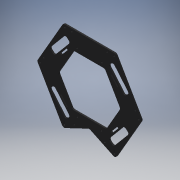
# Autodesk Inventor part: Bottom Plate
Saved by Autodesk Inventor 2017 (Build 210142000, 142)
## iProperties
Created: 2016-10-01
Part Number: Bottom Plate
Material: PVC, Unplasticized
Document SubType Name: Modeling
Designer: James Yelland
Density: 1.29 g/cm^3
Appearance: Smooth - White
Mass: 37.5584 g
Surface Area: 327.952 cm^2
Volume: 29.115 cm^3
Author: James Yelland
Autodesk Inventor part; units mm, degrees
ref_plane "YZ Plane" through (0, 0, 0) normal (1, 0, 0) x (0, 1, 0)
ref_plane "XZ Plane" through (0, 0, 0) normal (0, 1, 0) x (-1, 0, 0)
ref_plane "XY Plane" through (0, 0, 0) normal (0, 0, 1) x (1, 0, 0)
sketch "Sketch1" plane through (0, 0, 0) normal (0, 1, 0) x (-1, 0, 0)
  line L0 (103.5566, -2.5) -> (54.8095, -86.9325)
  line L1 (-54.8095, -86.9325) -> (-103.5566, -2.5)
  line L2 (-103.5566, 2.5) -> (-53.9434, 88.4327)
  line L3 (-49.6132, 90.9327) -> (49.6132, 90.9327)
  line L4 (53.9434, 88.4327) -> (103.5566, 2.5)
  line L5 (2.1497, -66.9563) -> (48.3297, -88.9468)
  line L6 (-2.1497, -66.9563) -> (-48.3297, -88.9468)
  arc A0 (48.3297, -88.9468) -> (54.8095, -86.9325) centre (50.4794, -84.4325) ccw
  arc A1 (2.1497, -66.9563) -> (-2.1497, -66.9563) centre (0, -71.4706) ccw
  arc A2 (-54.8095, -86.9325) -> (-48.3297, -88.9468) centre (-50.4794, -84.4325) ccw
  arc A3 (-103.5566, 2.5) -> (-103.5566, -2.5) centre (-99.2265, 0) ccw
  arc A4 (-49.6132, 90.9327) -> (-53.9434, 88.4327) centre (-49.6132, 85.9327) ccw
  arc A5 (53.9434, 88.4327) -> (49.6132, 90.9327) centre (49.6132, 85.9327) ccw
  arc A6 (103.5566, -2.5) -> (103.5566, 2.5) centre (99.2265, 0) ccw
  circle A7 centre (49.6132, 85.9327) radius 1.6
  circle A8 centre (-49.6132, 85.9327) radius 1.6
  circle A9 centre (-99.2265, 0) radius 1.6
  circle A10 centre (99.2265, 0) radius 1.6
  circle A11 centre (-25, 62.282) radius 1.6
  circle A12 centre (25, 62.282) radius 1.6
  circle A13 centre (24, -57.282) radius 1.6
  circle A14 centre (-24, -57.282) radius 1.6
  circle A15 centre (-30.6147, -73.9104) radius 1.6
  circle A16 centre (30.6147, -73.9104) radius 1.6
  circle A17 centre (35.5991, 85.9437) radius 1.6
  circle A18 centre (-35.5945, 85.9327) radius 1.6
  circle A19 centre (92.2171, 12.1406) radius 1.6
  circle A20 centre (-92.2171, 12.1406) radius 1.6
  arc A21 (31.3397, -49.282) -> (35.6699, -46.782) centre (31.3397, -44.282) ccw
  line L7 (31.3397, -49.282) -> (-31.3397, -49.282)
  arc A22 (-35.6699, -46.782) -> (-31.3397, -49.282) centre (-31.3397, -44.282) ccw
  line L8 (-35.6699, -46.782) -> (-61.2361, -2.5)
  arc A23 (-61.2361, 2.5) -> (-61.2361, -2.5) centre (-56.906, 0) ccw
  line L9 (-61.2361, 2.5) -> (-32.7831, 51.782)
  arc A24 (-28.453, 54.282) -> (-32.7831, 51.782) centre (-28.453, 49.282) ccw
  line L10 (-28.453, 54.282) -> (28.453, 54.282)
  arc A25 (32.7831, 51.782) -> (28.453, 54.282) centre (28.453, 49.282) ccw
  line L11 (32.7831, 51.782) -> (61.2361, 2.5)
  arc A26 (61.2361, -2.5) -> (61.2361, 2.5) centre (56.906, 0) ccw
  line L12 (61.2361, -2.5) -> (35.6699, -46.782)
  arc A27 (67.8361, 29.5077) -> (73.4714, 29.0147) centre (70.9003, 32.0789) ccw
  arc A28 (77.3017, 32.2286) -> (77.7947, 37.8639) centre (74.7305, 35.2928) ccw
  line L13 (73.4714, 29.0147) -> (77.3017, 32.2286)
  arc A29 (50.7976, 70.0378) -> (45.1623, 70.5308) centre (47.7335, 67.4666) ccw
  line L14 (45.1623, 70.5308) -> (41.3321, 67.3169)
  arc A30 (41.3321, 67.3169) -> (40.8391, 61.6815) centre (43.9032, 64.2527) ccw
  line L15 (64.2962, 53.9509) -> (50.7976, 70.0378)
  line L16 (64.2962, 53.9509) -> (77.7947, 37.8639)
  line L17 (40.8391, 61.6815) -> (67.8361, 29.5077)
  line L18 (49.7796, 41.77) -> (43.3517, 49.4305)
  line L19 (43.3517, 49.4305) -> (45.6499, 51.3589)
  line L20 (45.6499, 51.3589) -> (58.5056, 36.038)
  line L21 (58.5056, 36.038) -> (56.2075, 34.1096)
  line L22 (56.2075, 34.1096) -> (49.7796, 41.77)
  arc A31 (73.4714, -29.0147) -> (67.8361, -29.5077) centre (70.9003, -32.0789) ccw
  line L23 (54.3376, -45.5946) -> (57.5515, -41.7644)
  line L24 (45.6499, -51.3589) -> (58.5056, -36.038)
  line L25 (58.5056, -36.038) -> (56.2075, -34.1096)
  line L26 (40.8391, -61.6815) -> (67.8361, -29.5077)
  line L27 (64.2962, -53.9509) -> (77.7947, -37.8639)
  line L28 (73.4714, -29.0147) -> (77.3017, -32.2286)
  arc A32 (77.7947, -37.8639) -> (77.3017, -32.2286) centre (74.7305, -35.2928) ccw
  line L29 (43.3517, -49.4305) -> (45.6499, -51.3589)
  line L30 (49.7796, -41.77) -> (43.3517, -49.4305)
  arc A33 (45.1623, -70.5308) -> (50.7976, -70.0378) centre (47.7335, -67.4666) ccw
  line L31 (64.2962, -53.9509) -> (50.7976, -70.0378)
  line L32 (45.1623, -70.5308) -> (41.3321, -67.3169)
  arc A34 (40.8391, -61.6815) -> (41.3321, -67.3169) centre (43.9032, -64.2527) ccw
  line L33 (56.2075, -34.1096) -> (49.7796, -41.77)
  line L34 (-40.8391, -61.6815) -> (-67.8361, -29.5077)
  arc A35 (-67.8361, -29.5077) -> (-73.4714, -29.0147) centre (-70.9003, -32.0789) ccw
  line L35 (-45.6499, -51.3589) -> (-58.5056, -36.038)
  line L36 (-64.2962, -53.9509) -> (-77.7947, -37.8639)
  line L37 (-73.4714, -29.0147) -> (-77.3017, -32.2286)
  arc A36 (-77.3017, -32.2286) -> (-77.7947, -37.8639) centre (-74.7305, -35.2928) ccw
  line L38 (-43.3517, -49.4305) -> (-45.6499, -51.3589)
  line L39 (-49.7796, -41.77) -> (-43.3517, -49.4305)
  line L40 (-56.2075, -34.1096) -> (-49.7796, -41.77)
  line L41 (-45.1623, -70.5308) -> (-41.3321, -67.3169)
  arc A37 (-50.7976, -70.0378) -> (-45.1623, -70.5308) centre (-47.7335, -67.4666) ccw
  line L42 (-64.2962, -53.9509) -> (-50.7976, -70.0378)
  arc A38 (-41.3321, -67.3169) -> (-40.8391, -61.6815) centre (-43.9032, -64.2527) ccw
  line L43 (-40.8391, 61.6815) -> (-67.8361, 29.5077)
  arc A39 (-73.4714, 29.0147) -> (-67.8361, 29.5077) centre (-70.9003, 32.0789) ccw
  line L44 (-73.4714, 29.0147) -> (-77.3017, 32.2286)
  arc A40 (-77.7947, 37.8639) -> (-77.3017, 32.2286) centre (-74.7305, 35.2928) ccw
  line L45 (-64.2962, 53.9509) -> (-77.7947, 37.8639)
  line L46 (-56.2075, 34.1096) -> (-49.7796, 41.77)
  line L47 (-49.7796, 41.77) -> (-43.3517, 49.4305)
  line L48 (-45.6499, 51.3589) -> (-58.5056, 36.038)
  line L49 (-58.5056, 36.038) -> (-56.2075, 34.1096)
  line L50 (-64.2962, 53.9509) -> (-50.7976, 70.0378)
  line L51 (-43.3517, 49.4305) -> (-45.6499, 51.3589)
  line L52 (-45.1623, 70.5308) -> (-41.3321, 67.3169)
  arc A41 (-45.1623, 70.5308) -> (-50.7976, 70.0378) centre (-47.7335, 67.4666) ccw
  arc A42 (-40.8391, 61.6815) -> (-41.3321, 67.3169) centre (-43.9032, 64.2527) ccw
  line L53 (51.9794, -77.4325) -> (51.9794, -85.4325)
  line L54 (51.9794, -85.4325) -> (48.9794, -85.4325)
  line L55 (48.9794, -85.4325) -> (48.9794, -77.4325)
  line L56 (48.9794, -77.4325) -> (51.9794, -77.4325)
  line L57 (-48.9794, -77.4325) -> (-48.9794, -85.4325)
  line L58 (-48.9794, -85.4325) -> (-51.9794, -85.4325)
  line L59 (-51.9794, -85.4325) -> (-51.9794, -77.4325)
  line L60 (-51.9794, -77.4325) -> (-48.9794, -77.4325)
  line L61 (-56.2075, -34.1096) -> (-58.5056, -36.038)
  point P0 (52.5, -90.9327)
  point P1 (-52.5, 90.9327)
  point P2 (52.5, 90.9327)
  point P3 (70.4073, 26.4435)
  point P4 (80.3658, 34.7998)
  point P5 (38.2679, 64.7457)
  point P6 (48.2265, 73.102)
  point P7 (54.3376, 45.5946)
  point P8 (57.5515, 41.7644)
  point P9 (70.4073, -26.4435)
  point P10 (48.2265, -73.102)
  point P11 (38.2679, -64.7457)
  point P12 (80.3658, -34.7998)
  point P13 (-70.4073, -26.4435)
  point P14 (-83.093, -27.663)
  point P15 (-48.2265, -73.102)
  point P16 (-70.4073, 26.4435)
  point P17 (-80.3658, 34.7998)
  point P18 (-48.2265, 73.102)
  point P19 (-38.2679, 64.7457)
  dimension "d11" = 360
  dimension "d30" = 360
  dimension "d90" = 360
  dimension "d136" = 360
  dimension "d167" = 8
  dimension "d168" = 3
  dimension "d169" = 8
  dimension "d170" = 3
  constraints: 124 end point, 58 point on circle, 49 centre point, 35 point on line, 6 coincident, 4 parallel, 2 perpendicular, 1 midpoint, 1 vertical
  measures "d167" distance of L53.start L53.end
  measures "d168" distance of L53.end L54.end
  measures "d169" distance of L57.start L57.end
  measures "d170" distance of L57.end L58.end
extrude "Extrusion1" add sketch "Sketch1" along normal blind 3
body "Solid1"
